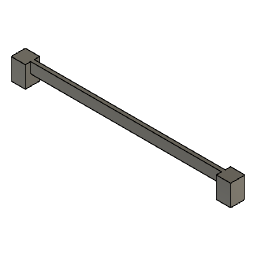
Target Stand v7 (Autodesk Fusion 360 archive; units mm, degrees)
design "Top of Stand"
Autodesk Fusion 360 part; units mm, degrees
sketch "Sketch1" plane through (0, 0, 0) normal (0, 0, 1) x (1, 0, 0)
  line L0 (68.9309, 100) -> (378.9309, 100)
  line L1 (378.9309, 100) -> (378.9309, 79.8)
  line L2 (378.9309, 79.8) -> (68.9309, 79.8)
  line L3 (68.9309, 79.8) -> (68.9309, 100)
  line L4 (73.9309, 95) -> (84.1309, 95)
  line L5 (84.1309, 95) -> (84.1309, 84.8)
  line L6 (84.1309, 84.8) -> (73.9309, 84.8)
  line L7 (73.9309, 84.8) -> (73.9309, 95)
  line L8 (89.1309, 100) -> (89.1309, 79.8)
  line L9 (363.7309, 95) -> (373.9309, 95)
  line L10 (373.9309, 95) -> (373.9309, 84.8)
  line L11 (373.9309, 84.8) -> (363.7309, 84.8)
  line L12 (363.7309, 84.8) -> (363.7309, 95)
  line L13 (358.7309, 100) -> (358.7309, 79.8)
  line L14 (89.1309, 92.4) -> (358.7309, 92.4)
  line L15 (358.7309, 92.4) -> (358.7309, 87.4)
  line L16 (358.7309, 87.4) -> (89.1309, 87.4)
  line L17 (89.1309, 87.4) -> (89.1309, 92.4)
  dimension "d1" = 310
  dimension "d2" = 20.2
  dimension "d3" = 20.2
  dimension "d4" = 5
  dimension "d5" = 5
  dimension "d6" = 5
  dimension "d7" = 5
  dimension "d8" = 20.2
  dimension "d9" = 20.2
  dimension "d10" = 5
  dimension "d11" = 5
  dimension "d12" = 5
  dimension "d13" = 5
  dimension "d14" = 5
  dimension "d15" = 7.6
  dimension "d16" = 7.6
  constraint horizontal L0
  constraint vertical L1
  constraint horizontal L2
  constraint vertical L3
  constraint horizontal L4
  constraint vertical L5
  constraint horizontal L6
  constraint vertical L7
  constraint coincident L0 L8.start
  constraint coincident L2 L8.end
  constraint perpendicular L2 L8
  constraint horizontal L9
  constraint vertical L10
  constraint horizontal L11
  constraint vertical L12
  constraint coincident L0 L13.start
  constraint coincident L2 L13.end
  constraint perpendicular L2 L13
  constraint horizontal L14
  constraint vertical L15
  constraint horizontal L16
  constraint vertical L17
  constraint coincident L13 L15.end
  constraint coincident L8 L14.start
  measures "d1" distance of L1 L3
  measures "d2" distance of L0.start L2.end
  measures "d3" distance of L3 L8
  measures "d4" distance of L5 L8
  measures "d5" distance of L0 L4
  measures "d6" distance of L3 L7
  measures "d7" distance of L2 L6
  measures "d8" distance of L0.end L1.end
  measures "d9" distance of L1 L13
  measures "d10" distance of L0 L9
  measures "d11" distance of L1 L10
  measures "d12" distance of L2 L11
  measures "d13" distance of L12 L13
  measures "d14" distance of L14 L16
  measures "d15" distance of L0 L14
  measures "d16" distance of L2 L16
extrude "Extrude1" add sketch "Sketch1" against normal blind 2.5 contours L4 L5 L6 L7 | L9 L10 L11 L12 makes body 1 at (367.1309, 91.6, 0) makes body 2 at (77.3309, 91.6, 0)
extrude "Extrude2" add sketch "Sketch1" against normal blind 30 contours L0 L2 L3 L8 L17 | L0 L1 L2 L13 L15 bodies 1 2
extrude "Extrude3" add sketch "Sketch1" against normal blind 15 contours L8 L13 L14 L15 L16 L17 bodies 1 2

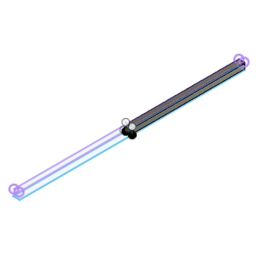
design "Picture Stand Poles"
Autodesk Fusion 360 part; units mm, degrees
sketch "Sketch1" plane through (0, 0, 0) normal (0, 0, 1) x (1, 0, 0)
  line L0 (-77.3846, -285.6532) -> (-87.3846, -285.6532)
  line L1 (-77.3846, 64.3468) -> (-77.3846, -285.6532)
  line L2 (-87.3846, -285.6532) -> (-87.3846, 64.3468)
  line L3 (-87.3846, 64.3468) -> (-77.3846, 64.3468)
  dimension "d11" = 10
  dimension "d12" = 350
  constraint horizontal L3
  constraint vertical L1
  constraint horizontal L0
  constraint vertical L2
  measures "d11" distance of L1.start L2.end
  measures "d12" distance of L2.end L0.end
extrude "Extrude3" add sketch "Sketch1" along normal blind 10
fillet "Fillet3" radius 1 2 edges at (-77.3846, -110.6532, 10) (-87.3846, -110.6532, 10)
fillet "Fillet4" radius 1 2 edges at (-77.3846, -110.6532, 0) (-87.3846, -110.6532, 0)
sketch "Sketch2" plane through (0, -285.6532, 0) normal (0, -1, 0) x (1, 0, 0)
  arc A0 (-87.3846, 1) -> (-86.3846, 0) centre (-86.3846, 1) ccw
  line L0 (-86.3846, 0) -> (-78.3846, 0)
  arc A1 (-78.3846, 0) -> (-77.3846, 1) centre (-78.3846, 1) ccw
  line L1 (-77.3846, 1) -> (-77.3846, 9)
  arc A2 (-77.3846, 9) -> (-78.3846, 10) centre (-78.3846, 9) ccw
  line L2 (-78.3846, 10) -> (-86.3846, 10)
  arc A3 (-86.3846, 10) -> (-87.3846, 9) centre (-86.3846, 9) ccw
  line L3 (-87.3846, 9) -> (-87.3846, 1)
  line L4 (-77.3846, 0, -175) -> (-77.3846, 7, -175)
  line L5 (-78.3846, 10, -350) -> (-78.3846, 10, 0)
  line L6 (-86.3846, 10, 0) -> (-86.3846, 10, -350)
  line L7 (-78.3846, 10, -175) -> (-86.3846, 10, -175)
  line L8 (-77.3846, 7, -175) -> (-77.3846, 11, -175)
  line L9 (-78.3846, 10, -175) -> (-77.3846, 10, -175)
  line L10 (-87.3846, 0, -175) -> (-90.5, 0, -175)
  line L11 (-87.3846, 0, -175) -> (-87.3846, 12, -175)
  line L12 (-86.3846, 10, -175) -> (-87.3846, 10, -175)
  line L13 (-87.3846, 0, -175) -> (-77.3846, 0, -175)
  point P0 (-77.3846, 0)
  point P1 (-87.3846, 0)
extrude "Extrude4" cut sketch "Sketch2" against normal blind 175

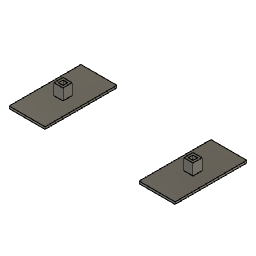
design "Base of Stand"
Autodesk Fusion 360 part; units mm, degrees
sketch "Sketch1" plane through (0, 0, 0) normal (0, 0, 1) x (1, 0, 0)
  line L0 (48.9309, 100) -> (358.9309, 100)
  line L1 (358.9309, 100) -> (358.9309, 79.8)
  line L2 (358.9309, 79.8) -> (48.9309, 79.8)
  line L3 (48.9309, 79.8) -> (48.9309, 100)
  line L4 (53.9309, 95) -> (64.1309, 95)
  line L5 (64.1309, 95) -> (64.1309, 84.8)
  line L6 (64.1309, 84.8) -> (53.9309, 84.8)
  line L7 (53.9309, 84.8) -> (53.9309, 95)
  line L8 (69.1309, 100) -> (69.1309, 79.8)
  line L9 (343.7309, 95) -> (353.9309, 95)
  line L10 (353.9309, 95) -> (353.9309, 84.8)
  line L11 (353.9309, 84.8) -> (343.7309, 84.8)
  line L12 (343.7309, 84.8) -> (343.7309, 95)
  line L13 (338.7309, 100) -> (338.7309, 79.8)
  line L14 (338.7309, 92.4) -> (338.7309, 87.4)
  line L15 (69.1309, 87.4) -> (69.1309, 92.4)
  line L16 (18.9309, 170) -> (99.1309, 170)
  line L17 (99.1309, 170) -> (99.1309, 9.8)
  line L18 (99.1309, 9.8) -> (18.9309, 9.8)
  line L19 (18.9309, 9.8) -> (18.9309, 170)
  line L20 (308.7309, 170) -> (388.9309, 170)
  line L21 (388.9309, 170) -> (388.9309, 9.8)
  line L22 (388.9309, 9.8) -> (308.7309, 9.8)
  line L23 (308.7309, 9.8) -> (308.7309, 170)
  dimension "d1" = 310
  dimension "d2" = 20.2
  dimension "d3" = 20.2
  dimension "d4" = 5
  dimension "d5" = 5
  dimension "d6" = 5
  dimension "d7" = 5
  dimension "d8" = 20.2
  dimension "d9" = 20.2
  dimension "d10" = 5
  dimension "d11" = 5
  dimension "d12" = 5
  dimension "d13" = 5
  dimension "d17" = 70
  dimension "d18" = 30
  dimension "d19" = 70
  dimension "d20" = 30
  dimension "d21" = 70
  dimension "d22" = 70
  dimension "d23" = 30
  dimension "d24" = 30
  constraint horizontal L0
  constraint vertical L1
  constraint horizontal L2
  constraint vertical L3
  constraint horizontal L4
  constraint vertical L5
  constraint horizontal L6
  constraint vertical L7
  constraint coincident L0 L8.start
  constraint coincident L2 L8.end
  constraint perpendicular L2 L8
  constraint horizontal L9
  constraint vertical L10
  constraint horizontal L11
  constraint vertical L12
  constraint coincident L0 L13.start
  constraint coincident L2 L13.end
  constraint perpendicular L2 L13
  constraint vertical L14
  constraint vertical L15
  constraint coincident L13 L14.end
  constraint coincident L8 L15.end
  constraint horizontal L16
  constraint vertical L17
  constraint horizontal L18
  constraint vertical L19
  constraint horizontal L20
  constraint vertical L21
  constraint horizontal L22
  constraint vertical L23
  measures "d1" distance of L1 L3
  measures "d2" distance of L0.start L2.end
  measures "d3" distance of L3 L8
  measures "d4" distance of L5 L8
  measures "d5" distance of L0 L4
  measures "d6" distance of L3 L7
  measures "d7" distance of L2 L6
  measures "d8" distance of L0.end L1.end
  measures "d9" distance of L1 L13
  measures "d10" distance of L0 L9
  measures "d11" distance of L1 L10
  measures "d12" distance of L2 L11
  measures "d13" distance of L12 L13
  measures "d17" distance of L0 L16
  measures "d18" distance of L8 L17
  measures "d19" distance of L2 L18
  measures "d20" distance of L3 L19
  measures "d21" distance of L0 L20
  measures "d22" distance of L2 L22
  measures "d23" distance of L1 L21
  measures "d24" distance of L13 L23
extrude "Extrude1" add sketch "Sketch1" along normal blind 2.5 contours L4 L5 L6 L7 | L9 L10 L11 L12 makes body 1 at (57.3309, 88.2, 0) makes body 2 at (347.1309, 91.6, 0)
extrude "Extrude2" add sketch "Sketch1" along normal blind 30 contours L0 L2 L3 L8 L15 | L0 L1 L2 L13 L14 bodies 1 2
extrude "Extrude3" add sketch "Sketch1" along normal blind 5 contours L0 L2 L3 L16 L17 L18 L19 | L0 L2 L8 L15 L17 | L0 L1 L2 L20 L21 L22 L23 | L0 L2 L13 L14 L23 bodies 1 2
